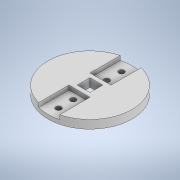
# Autodesk Inventor part: prop_base
Saved by Autodesk Inventor 2021 (Build 250183000, 183)
## iProperties
Created: 2020-08-19
Part Number: prop_base
Material: Generic
Document SubType Name: Modeling
Designer: elizabethhassan
Density: 1 g/cm^3
Appearance: Default
Mass: 4.24228 g
Surface Area: 31.7615 cm^2
Volume: 4.24228 cm^3
Author: elizabethhassan
Autodesk Inventor part; units mm, degrees
ref_plane "YZ Plane" through (0, 0, 0) normal (1, 0, 0) x (0, 1, 0)
ref_plane "XZ Plane" through (0, 0, 0) normal (0, 1, 0) x (-1, 0, 0)
sketch "Sketch1" plane through (0, 0, 0) normal (0, 1, 0) x (-1, 0, 0)
  circle A0 centre (0, 0) radius 20
  dimension "d0" = 40
  constraints: 1 centre point, 1 coincident
  measures "d0" diameter of A0
extrude "Extrusion1" add sketch "Sketch1" along normal blind 6
sketch "Sketch3" plane through (0, 6, 0) normal (0, 1, 0) x (1, 0, 0)
  line L0 (0, 0) -> (0, 20)
  circle A0 centre (0, 0) radius 20 projected
  line L1 (5, 35) -> (5, 5)
  line L2 (5, 5) -> (-5, 5)
  line L3 (-5, 5) -> (-5, 35)
  line L4 (-5, 35) -> (5, 35)
  line L5 (5, 35) -> (-5, 5) construction
  line L6 (5, 5) -> (-5, 35) construction
  line L7 (20, 0) -> (-20, 0) construction
  line L8 (5, -35) -> (5, -5)
  line L9 (5, -5) -> (-5, -5)
  line L10 (-5, -5) -> (-5, -35)
  line L11 (-5, -35) -> (5, -35)
  point P0 (-5, 19.3649)
  point P1 (5, 19.3649)
  point P2 (-5, -19.3649)
  point P3 (5, -19.3649)
  dimension "d11" = 30
  dimension "d12" = 10
  constraints: 24 end point, 4 symmetric about line, 3 point on circle, 2 midpoint, 2 parallel, 1 horizontal, 1 perpendicular, 1 vertical
  measures "d11" distance of L1.start L1.end
  measures "d12" distance of L1.end L2.end
extrude "Extrusion2" cut sketch "Sketch3" against normal blind 2 contours L2 L3 A0 L0 | L0 A0 L1 L2 | L10 L9 L8 A0
sketch "Sketch5" plane through (0, 4, 0) normal (0, 1, 0) x (1, 0, 0)
  circle A0 centre (0, -8) radius 1
  circle A1 centre (0, -15) radius 1
  line L0 (-5, -5) -> (5, -5) projected
  arc A2 (-5, 19.3649) -> (-5, -19.3649) centre (0, 0) ccw projected
  line L1 (-20, 0) -> (20, 0) construction
  arc A3 (5, -19.3649) -> (5, 19.3649) centre (0, 0) ccw projected
  circle A4 centre (0, 8) radius 1
  circle A5 centre (0, 15) radius 1
  line L2 (-28, 0) -> (28, 0) projected
  line L3 (-5, 5) -> (-5, 19.3649) projected
  dimension "d20" = 2
  dimension "d21" = 2
  dimension "d42" = 8
  dimension "d43" = 7
  dimension "d44" = 8
  dimension "d45" = 20
  dimension "d47" = 5
  constraints: 4 centre point, 2 end point, 2 point on circle, 2 symmetric about line, 1 horizontal, 2 other
  measures "d20" diameter of A0
  measures "d21" diameter of A1
  measures "d42" distance from line of A0.centre L2
  measures "d43" distance of A0.centre A1.centre
  measures "d44" distance from line of L2 A4.centre
  measures "d45" distance from line of A5.centre L0
  measures "d47" distance from line of L3 A5.centre
hole "Hole2" at (0, 4, 15) at (0, 4, 8) at (0, 4, -8) at (0, 4, -15) direction (0, -1, 0) diameter 2.6416 depth 10.979 tip angle 118 thread size "6-32 UNC" class "2B" standard "ANSI Unified Screw Threads"
sketch "Sketch6" plane through (0, 6, 0) normal (0, 1, 0) x (1, 0, 0)
  line L0 (3.05, 3.05) -> (-3.05, 3.05)
  line L1 (-3.05, 3.05) -> (-3.05, -3.05)
  line L2 (-3.05, -3.05) -> (3.05, -3.05)
  line L3 (3.05, -3.05) -> (3.05, 3.05)
  point P0 (0, 0)
  dimension "d31" = 6.1
  dimension "d32" = 6.1
  dimension "d33" = 3.05
  dimension "d34" = 3.05
  constraints: 8 end point, 2 parallel, 1 horizontal, 1 perpendicular
  measures "d31" distance of L2.end L1.end
  measures "d32" distance of L1.end L0.end
  measures "d33" distance from line of point (0, 0) L0
  measures "d34" distance from line of L3 point (0, 0)
extrude "Extrusion4" cut sketch "Sketch6" against normal blind 10
ref_plane "Work Plane1" through (0, 0, 20) normal (0, 0, 1) x (1, 0, 0)
sketch "Sketch7" plane through (0, 0, 20) normal (0, 0, 1) x (1, 0, 0)
  line L0 (20, 0) -> (-20, 0) projected
  line L1 (-20, 0) -> (20, 0)
  line L2 (20, 0) -> (20, 2)
  line L3 (20, 2) -> (-20, 2)
  line L4 (-20, 2) -> (-20, 0)
  point P0 (0, 0)
  dimension "d38" = 40
  dimension "d39" = 2
  constraints: 8 end point, 2 parallel, 1 horizontal, 1 perpendicular
  measures "d38" distance of L3.end L2.end
  measures "d39" distance of L2.end L1.end
extrude "Extrusion5" cut sketch "Sketch7" against normal blind 40
sketch "Sketch8" plane through (0, 6, 0) normal (0, 1, 0) x (1, 0, 0)
  line L0 (-20, -20) -> (-7, -20)
  line L1 (-7, -20) -> (-7, 20)
  line L2 (-7, 20) -> (-20, 20)
  line L3 (-20, 20) -> (-20, -20)
  line L4 (7, -20) -> (20, -20)
  line L5 (20, -20) -> (20, 20)
  line L6 (20, 20) -> (7, 20)
  line L7 (7, 20) -> (7, -20)
  line L8 (5, 19.3649) -> (5, 5) projected
  line L9 (-5, 5) -> (-5, 19.3649) projected
  line L10 (28.233, -20) -> (-28.0388, -20) projected
  point P0 (0, 0)
  dimension "d48" = 40
  dimension "d49" = 0
  dimension "d50" = 0
  dimension "d51" = 2
  dimension "d52" = 2
  dimension "d53" = 0
  dimension "d54" = 13
  dimension "d55" = 13
  constraints: 16 end point, 4 parallel, 2 horizontal, 2 perpendicular
  measures "d48" distance of L2.end L0.start
  measures "d49" distance between parallel lines of L0 L4
  measures "d50" distance between parallel lines of L2 L6
  measures "d51" distance between parallel lines of L8 L7
  measures "d52" distance between parallel lines of L9 L1
  measures "d53" distance between parallel lines of L10 L4
  measures "d54" distance of L0.start L0.end
  measures "d55" distance of L5.end L6.end
body "Solid1"
